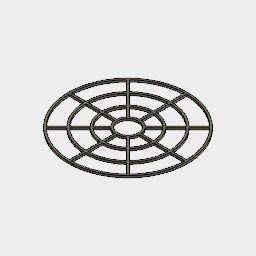
290mm_calibration_spiderweb (Autodesk Fusion 360 design; units mm, degrees)
Autodesk Fusion 360 part; units mm, degrees
sketch "Sketch1" plane through (0, 0, 0) normal (0, 1, 0) x (1, 0, 0)
  circle A0 centre (0, 0) radius 145
  circle A1 centre (0, 0) radius 140
  circle A2 centre (0, 0) radius 25
  circle A3 centre (0, 0) radius 30
  line L0 (-2.5, 140) -> (-2.5, 29.8957)
  line L1 (2.5, 140) -> (2.5, 29.8957)
  circle A4 centre (0, 0) radius 105
  circle A5 centre (0, 0) radius 100
  circle A6 centre (0, 0) radius 65
  circle A7 centre (0, 0) radius 60
  line L2 (-97.2272, 100.7627) -> (-19.3717, 22.9072)
  line L3 (-100.7627, 97.2272) -> (-22.9072, 19.3717)
  line L4 (-140, 2.5) -> (-29.8957, 2.5)
  line L5 (-140, -2.5) -> (-29.8957, -2.5)
  line L6 (-100.7627, -97.2272) -> (-22.9072, -19.3717)
  line L7 (-97.2272, -100.7627) -> (-19.3717, -22.9072)
  line L8 (-2.5, -140) -> (-2.5, -29.8957)
  line L9 (2.5, -140) -> (2.5, -29.8957)
  line L10 (97.2272, -100.7627) -> (19.3717, -22.9072)
  line L11 (100.7627, -97.2272) -> (22.9072, -19.3717)
  line L12 (140, -2.5) -> (29.8957, -2.5)
  line L13 (140, 2.5) -> (29.8957, 2.5)
  line L14 (100.7627, 97.2272) -> (22.9072, 19.3717)
  line L15 (97.2272, 100.7627) -> (19.3717, 22.9072)
  dimension "d1" = 290
  dimension "d2" = 280
  dimension "d3" = 50
  dimension "d4" = 60
  dimension "d7" = 210
  dimension "d8" = 130
  dimension "d10" = 360
  measures "d1" diameter of A0
  measures "d2" diameter of A1
  measures "d3" diameter of A2
  measures "d4" diameter of A3
  measures "d7" diameter of A4
  measures "d8" diameter of A6
extrude "Extrude1" add sketch "Sketch1" along normal blind 5 contours A0 | A1 A4 L12 L13 | A1 A4 L14 L15 | A4 A5 L13 L14 | A4 A5 L12 L13 | A1 A4 L10 L11 | A4 A5 L11 L12 | A4 A5 L14 L15 | A5 A6 L12 L13 | A4 A5 L10 L11 | A1 L0 L1 A4 | L1 A4 A5 L15 | A5 A6 L14 L15 | A6 A7 L13 L14 | A6 A7 L12 L13 | A1 A4 L8 L9 | A4 A5 L9 L10 | A5 A6 L10 L11 | A6 A7 L11 L12 | L0 L1 A4 A5 | A6 A7 L14 L15 | A3 A7 L12 L13 | A4 A5 L8 L9 | A6 A7 L10 L11 | A1 A4 L2 L3 | L0 A4 A5 L2 | L0 L1 A5 A6 | L1 A6 A7 L15 | A3 A7 L14 L15 | A3 | A1 A4 L6 L7 | A4 A5 L7 L8 | A5 A6 L8 L9 | A6 A7 L9 L10 | A3 A7 L10 L11 | A4 A5 L2 L3 | L0 L1 A6 A7 | A4 A5 L6 L7 | A6 A7 L8 L9 | A1 A4 L4 L5 | A4 A5 L3 L4 | A5 A6 L2 L3 | L0 A6 A7 L2 | A3 L0 L1 A7 | A4 A5 L5 L6 | A5 A6 L6 L7 | A6 A7 L7 L8 | A3 A7 L8 L9 | A4 A5 L4 L5 | A6 A7 L2 L3 | A6 A7 L6 L7 | A5 A6 L4 L5 | A6 A7 L3 L4 | A3 A7 L2 L3 | A6 A7 L5 L6 | A3 A7 L6 L7 | A6 A7 L4 L5 | A3 A7 L4 L5
